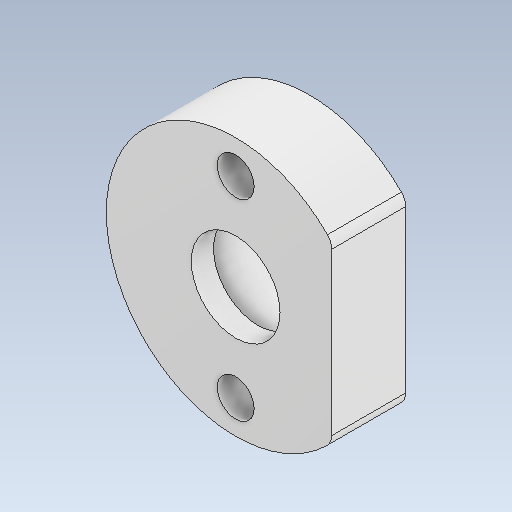
# Autodesk Inventor part: 0008-10-034 Suport_Rulment
Saved by Autodesk Inventor 2020 (Build 240168000, 168)
## iProperties
Created: 2021-02-03
Part Number: 0008-10-034 Suport_Rulment
Material: ABS Plastic
Document SubType Name: Modeling
Designer: Iulian Bors
Density: 1.06 g/cm^3
Appearance: Smooth - White
Mass: 7.10581 g
Surface Area: 33.3585 cm^2
Volume: 6.7036 cm^3
Description: Suport Rulment
Author: Iulian Bors
Subject: 034
Autodesk Inventor part; units mm, degrees
ref_plane "YZ Plane" through (0, 0, 0) normal (1, 0, 0) x (0, 1, 0)
ref_plane "XZ Plane" through (0, 0, 0) normal (0, 1, 0) x (-1, 0, 0)
ref_plane "XY Plane" through (0, 0, 0) normal (0, 0, 1) x (1, 0, 0)
sketch "Sketch1" plane through (0, 0, 0) normal (0, 0, 1) x (1, 0, 0)
  circle A0 centre (0, 0) radius 6
  circle A1 centre (0, 0) radius 17.5
  dimension "d0" = 12
  dimension "d1" = 35
  constraints: 2 centre point, 2 coincident
  measures "d0" diameter of A0
  measures "d1" diameter of A1
extrude "Extrusion1" add sketch "Sketch1" along normal blind 10
sketch "Sketch4" plane through (0, 0, 0) normal (0, 0, -1) x (-1, 0, 0)
  circle A0 centre (0, 0) radius 13 construction
  point P0 (0, -13)
  point P1 (0, 13)
  dimension "d7" = 26
  constraints: 2 point on circle, 2 vertical alignment, 1 centre point, 1 coincident
  measures "d7" diameter of A0
hole "Hole1" at (0, -13, 0) at (0, 13, 0) direction (0, 0, 1) diameter 5 end through all
sketch "Sketch5" plane through (0, 0, 0) normal (0, 0, -1) x (-1, 0, 0)
  circle A0 centre (0, 0) radius 8.15
  dimension "d15" = 16.3
  constraints: 1 centre point, 1 coincident
  measures "d15" diameter of A0
extrude "Extrusion3" cut sketch "Sketch5" against normal blind 7
sketch "Sketch6" plane through (0, 0, 10) normal (0, 0, 1) x (1, 0, 0)
  line L0 (13, -11.7154) -> (13, 11.7154)
  circle A0 centre (0, 0) radius 17.5 projected
  circle A1 centre (0, -13) radius 2.5 construction
  circle A2 centre (0, 13) radius 2.5 construction
  line L1 (0, -13) -> (0, 13) construction
  dimension "d22" = 13
  constraints: 4 end point, 2 point on circle, 1 parallel, 1 vertical
  measures "d22" distance from line of A0.centre L0
extrude "Extrusion4" cut sketch "Sketch6" against normal through all contours L0 A0 picked at (13.8164, -2.7401)
fillet "Fillet2" radius 2 2 edges at (13, -11.7154, 5) (13, 11.7154, 5)
body "Solid1"
